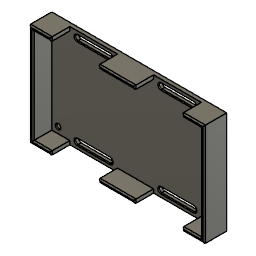
power_tray_v0_1_fusion_final (Autodesk Fusion 360 design; units mm, degrees)
part number: 2026-05-26-08-43-21-523
Autodesk Fusion 360 part; units mm, degrees
sketch "草图12" plane through (0, 0, 0) normal (0, 0, 1) x (1, 0, 0)
  line L0 (-69.75, -40.85) -> (69.75, -40.85)
  line L1 (69.75, -40.85) -> (69.75, 40.85)
  line L2 (69.75, 40.85) -> (-69.75, 40.85)
  line L3 (-69.75, 40.85) -> (-69.75, -40.85)
extrude "拉伸12" add sketch "草图12" along normal blind 3
ref_plane "工作平面2" through (0, 0, 3) normal (0, 0, 1) x (1, 0, 0)
sketch "草图13" plane through (0, 0, 3) normal (0, 0, 1) x (1, 0, 0)
  line L0 (-69.75, -40.85) -> (-66.75, -40.85)
  line L1 (-66.75, -40.85) -> (-66.75, 40.85)
  line L2 (-66.75, 40.85) -> (-69.75, 40.85)
  line L3 (-69.75, 40.85) -> (-69.75, -40.85)
extrude "拉伸13" add sketch "草图13" along normal blind 15
sketch "草图14" plane through (0, 0, 3) normal (0, 0, 1) x (1, 0, 0)
  line L0 (66.75, -40.85) -> (69.75, -40.85)
  line L1 (69.75, -40.85) -> (69.75, 40.85)
  line L2 (69.75, 40.85) -> (66.75, 40.85)
  line L3 (66.75, 40.85) -> (66.75, -40.85)
extrude "拉伸14" add sketch "草图14" along normal blind 15
sketch "草图15" plane through (0, 0, 3) normal (0, 0, 1) x (1, 0, 0)
  line L0 (-66.75, -40.85) -> (-52.375, -40.85)
  line L1 (-52.375, -40.85) -> (-52.375, -37.85)
  line L2 (-52.375, -37.85) -> (-66.75, -37.85)
  line L3 (-66.75, -37.85) -> (-66.75, -40.85)
extrude "拉伸15" add sketch "草图15" along normal blind 15
sketch "草图16" plane through (0, 0, 3) normal (0, 0, 1) x (1, 0, 0)
  line L0 (-14.375, -40.85) -> (14.375, -40.85)
  line L1 (14.375, -40.85) -> (14.375, -37.85)
  line L2 (14.375, -37.85) -> (-14.375, -37.85)
  line L3 (-14.375, -37.85) -> (-14.375, -40.85)
extrude "拉伸16" add sketch "草图16" along normal blind 15
sketch "草图17" plane through (0, 0, 3) normal (0, 0, 1) x (1, 0, 0)
  line L0 (52.375, -40.85) -> (66.75, -40.85)
  line L1 (66.75, -40.85) -> (66.75, -37.85)
  line L2 (66.75, -37.85) -> (52.375, -37.85)
  line L3 (52.375, -37.85) -> (52.375, -40.85)
extrude "拉伸17" add sketch "草图17" along normal blind 15
sketch "草图18" plane through (0, 0, 3) normal (0, 0, 1) x (1, 0, 0)
  line L0 (-66.75, 37.85) -> (-52.375, 37.85)
  line L1 (-52.375, 37.85) -> (-52.375, 40.85)
  line L2 (-52.375, 40.85) -> (-66.75, 40.85)
  line L3 (-66.75, 40.85) -> (-66.75, 37.85)
extrude "拉伸18" add sketch "草图18" along normal blind 15
sketch "草图19" plane through (0, 0, 3) normal (0, 0, 1) x (1, 0, 0)
  line L0 (-14.375, 37.85) -> (14.375, 37.85)
  line L1 (14.375, 37.85) -> (14.375, 40.85)
  line L2 (14.375, 40.85) -> (-14.375, 40.85)
  line L3 (-14.375, 40.85) -> (-14.375, 37.85)
extrude "拉伸19" add sketch "草图19" along normal blind 15
sketch "草图20" plane through (0, 0, 3) normal (0, 0, 1) x (1, 0, 0)
  line L0 (52.375, 37.85) -> (66.75, 37.85)
  line L1 (66.75, 37.85) -> (66.75, 40.85)
  line L2 (66.75, 40.85) -> (52.375, 40.85)
  line L3 (52.375, 40.85) -> (52.375, 37.85)
extrude "拉伸20" add sketch "草图20" along normal blind 15
sketch "草图21" plane through (0, 0, 3) normal (0, 0, 1) x (1, 0, 0)
  line L0 (-46.375, -33.85) -> (-20.375, -33.85)
  line L1 (-20.375, -37.85) -> (-46.375, -37.85)
  arc A0 (-20.375, -37.85) -> (-20.375, -33.85) centre (-20.375, -35.85) ccw
  arc A1 (-46.375, -33.85) -> (-46.375, -37.85) centre (-46.375, -35.85) ccw
  line L2 (-46.375, 37.85) -> (-20.375, 37.85)
  line L3 (-20.375, 33.85) -> (-46.375, 33.85)
  arc A2 (-20.375, 33.85) -> (-20.375, 37.85) centre (-20.375, 35.85) ccw
  arc A3 (-46.375, 37.85) -> (-46.375, 33.85) centre (-46.375, 35.85) ccw
  line L4 (20.375, -33.85) -> (46.375, -33.85)
  line L5 (46.375, -37.85) -> (20.375, -37.85)
  arc A4 (46.375, -37.85) -> (46.375, -33.85) centre (46.375, -35.85) ccw
  arc A5 (20.375, -33.85) -> (20.375, -37.85) centre (20.375, -35.85) ccw
  line L6 (20.375, 37.85) -> (46.375, 37.85)
  line L7 (46.375, 33.85) -> (20.375, 33.85)
  arc A6 (46.375, 33.85) -> (46.375, 37.85) centre (46.375, 35.85) ccw
  arc A7 (20.375, 37.85) -> (20.375, 33.85) centre (20.375, 35.85) ccw
extrude "拉伸21" cut sketch "草图21" against normal blind 3.2
sketch "草图22" plane through (0, 0, 3) normal (0, 0, 1) x (1, 0, 0)
  circle A0 centre (-61.75, -32.85) radius 1.6
  circle A1 centre (-61.75, 32.85) radius 1.6
  circle A2 centre (61.75, -32.85) radius 1.6
  circle A3 centre (61.75, 32.85) radius 1.6
extrude "拉伸22" cut sketch "草图22" against normal blind 3.2
fillet "圆角2" radius 1 24 edges at (59.5625, 37.85, 18) (52.375, 39.35, 18) (66.75, 0, 18) (14.375, 39.35, 18) (0, 37.85, 18) (-14.375, 39.35, 18) (0, 40.85, 18) (-52.375, 39.35, 18) (-59.5625, 37.85, 18) (59.5625, -37.85, 18) (52.375, -39.35, 18) (0, -37.85, 18) (14.375, -39.35, 18) (-14.375, -39.35, 18) (0, -40.85, 18) (-59.5625, -37.85, 18) (-52.375, -39.35, 18) (-66.75, 0, 18) (61.0625, -40.85, 18) (69.75, 0, 18) (61.0625, 40.85, 18) (-69.75, 0, 18) (-61.0625, -40.85, 18) (-61.0625, 40.85, 18)
fillet "圆角3" radius 0.6 68 edges at (60.2583, -32.2714, 3) (-63.2417, 33.4286, 3) (-63.2417, -32.2714, 3) (60.2583, 33.4286, 3) (33.375, -37.85, 3) (18.375, -35.85, 3) (33.375, -33.85, 3) (48.375, -35.85, 3) (48.375, -35.85, 3) (33.375, -37.85, 3) (18.375, -35.85, 3) (33.375, -33.85, 3) (33.375, -33.85, 3) (48.375, -35.85, 3) (33.375, -37.85, 3) (18.375, -35.85, 3) (18.375, -35.85, 3) (33.375, -33.85, 3) (48.375, -35.85, 3) (33.375, -37.85, 3) (-33.375, 33.85, 3) (-48.375, 35.85, 3) (-33.375, 37.85, 3) (-18.375, 35.85, 3) (-18.375, 35.85, 3) (-33.375, 33.85, 3) (-48.375, 35.85, 3) (-33.375, 37.85, 3) (-33.375, 37.85, 3) (-18.375, 35.85, 3) (-33.375, 33.85, 3) (-48.375, 35.85, 3) (-48.375, 35.85, 3) (-33.375, 37.85, 3) (-18.375, 35.85, 3) (-33.375, 33.85, 3) (-33.375, -37.85, 3) (-48.375, -35.85, 3) (-33.375, -33.85, 3) (-18.375, -35.85, 3) (-18.375, -35.85, 3) (-33.375, -37.85, 3) (-48.375, -35.85, 3) (-33.375, -33.85, 3) (-33.375, -33.85, 3) (-18.375, -35.85, 3) (-33.375, -37.85, 3) (-48.375, -35.85, 3) (-48.375, -35.85, 3) (-33.375, -33.85, 3) (-18.375, -35.85, 3) (-33.375, -37.85, 3) (33.375, 33.85, 3) (18.375, 35.85, 3) (33.375, 37.85, 3) (48.375, 35.85, 3) (48.375, 35.85, 3) (33.375, 33.85, 3) (18.375, 35.85, 3) (33.375, 37.85, 3) (33.375, 37.85, 3) (48.375, 35.85, 3) (33.375, 33.85, 3) (18.375, 35.85, 3) (18.375, 35.85, 3) (33.375, 37.85, 3) (48.375, 35.85, 3) (33.375, 33.85, 3)
sketch "草图7" plane through (0, 0, 3) normal (0, 0, 1) x (1, 0, 0)
  line L0 (-66.75, 37.85) -> (-52.375, 37.85)
  line L1 (-52.375, 37.85) -> (-52.375, 40.85)
  line L2 (-52.375, 40.85) -> (-66.75, 40.85)
  line L3 (-66.75, 40.85) -> (-66.75, 37.85)
sketch "草图8" plane through (0, 0, 3) normal (0, 0, 1) x (1, 0, 0)
  line L0 (-14.375, 37.85) -> (14.375, 37.85)
  line L1 (14.375, 37.85) -> (14.375, 40.85)
  line L2 (14.375, 40.85) -> (-14.375, 40.85)
  line L3 (-14.375, 40.85) -> (-14.375, 37.85)
sketch "草图9" plane through (0, 0, 3) normal (0, 0, 1) x (1, 0, 0)
  line L0 (52.375, 37.85) -> (66.75, 37.85)
  line L1 (66.75, 37.85) -> (66.75, 40.85)
  line L2 (66.75, 40.85) -> (52.375, 40.85)
  line L3 (52.375, 40.85) -> (52.375, 37.85)
sketch "草图10" plane through (0, 0, 3) normal (0, 0, 1) x (1, 0, 0)
  line L0 (-46.375, -33.85) -> (-20.375, -33.85)
  line L1 (-20.375, -37.85) -> (-46.375, -37.85)
  arc A0 (-20.375, -37.85) -> (-20.375, -33.85) centre (-20.375, -35.85) ccw
  arc A1 (-46.375, -33.85) -> (-46.375, -37.85) centre (-46.375, -35.85) ccw
  line L2 (-46.375, 37.85) -> (-20.375, 37.85)
  line L3 (-20.375, 33.85) -> (-46.375, 33.85)
  arc A2 (-20.375, 33.85) -> (-20.375, 37.85) centre (-20.375, 35.85) ccw
  arc A3 (-46.375, 37.85) -> (-46.375, 33.85) centre (-46.375, 35.85) ccw
  line L4 (20.375, -33.85) -> (46.375, -33.85)
  line L5 (46.375, -37.85) -> (20.375, -37.85)
  arc A4 (46.375, -37.85) -> (46.375, -33.85) centre (46.375, -35.85) ccw
  arc A5 (20.375, -33.85) -> (20.375, -37.85) centre (20.375, -35.85) ccw
  line L6 (20.375, 37.85) -> (46.375, 37.85)
  line L7 (46.375, 33.85) -> (20.375, 33.85)
  arc A6 (46.375, 33.85) -> (46.375, 37.85) centre (46.375, 35.85) ccw
  arc A7 (20.375, 37.85) -> (20.375, 33.85) centre (20.375, 35.85) ccw
sketch "草图11" plane through (0, 0, 3) normal (0, 0, 1) x (1, 0, 0)
  circle A0 centre (-61.75, -32.85) radius 1.6
  circle A1 centre (-61.75, 32.85) radius 1.6
  circle A2 centre (61.75, -32.85) radius 1.6
  circle A3 centre (61.75, 32.85) radius 1.6
named bodies: "power_tray_body"
